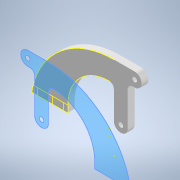
# Autodesk Inventor part: hinge
Saved by Autodesk Inventor 2020 (Build 240168000, 168)
## iProperties
Created: 2020-07-26
Part Number: hinge
Material: Generic
Document SubType Name: Modeling
Designer: Aarya
Density: 1 g/cm^3
Appearance: Default
Author: Aarya
Autodesk Inventor part; units mm, degrees
ref_plane "YZ Plane" through (0, 0, 0) normal (1, 0, 0) x (0, 1, 0)
ref_plane "XZ Plane" through (0, 0, 0) normal (0, 1, 0) x (-1, 0, 0)
ref_plane "XY Plane" through (0, 0, 0) normal (0, 0, 1) x (1, 0, 0)
sketch "Sketch1" plane through (0, 0, 0) normal (0, 0, 1) x (1, 0, 0)
  arc A0 (0, 18) -> (-18, 0.0024) centre (0, 0) ccw
  line L0 (0, 0) -> (0, -6.19)
  line L1 (0, -6.19) -> (2, -6.19)
  arc A1 (2, 30) -> (-33.6563, 0.0024) centre (2, -6.19) ccw
  line L2 (-33.6563, 0.0024) -> (-18, 0.0024)
  line L3 (3, 0) -> (3, 0)
  line L4 (6, 0) -> (32.7783, 0) construction
  line L5 (-33.6563, 0.0024) -> (-33.6563, 30.0024)
  line L6 (2, 30) -> (11, 30)
  line L7 (2, 30) -> (11, 30) construction
  line L8 (0, 0) -> (0, 3)
  line L9 (3, 3) -> (3, 3)
  line L10 (0, 3) -> (2, 3)
  line L11 (2, 6) -> (2, 16)
  line L12 (5, 3) -> (5, 3)
  line L13 (8, 6) -> (8, 22)
  arc A2 (2, 6) -> (5, 3) centre (5, 6) ccw
  arc A3 (5, 3) -> (8, 6) centre (5, 6) ccw
  arc A4 (2, 16) -> (0, 18) centre (0, 16) ccw
  arc A5 (11, 24) -> (11, 30) centre (11, 27) ccw
  line L14 (11, 24) -> (10, 24)
  arc A6 (10, 24) -> (8, 22) centre (10, 22) ccw
  circle A7 centre (5, 6) radius 1
  circle A8 centre (11, 27) radius 1
  line L15 (-33.6563, 0.0024) -> (-31.6563, 0.0024)
  line L16 (-27.1563, 0.0024) -> (-25.1563, 0.0024)
  point P0 (8, 3)
  point P1 (8, 24)
  point P2 (2, 17.8885)
  point P3 (-20.6563, 0.0024)
  dimension "d0" = 36
  dimension "d1" = 6.19
  dimension "d2" = 2
  dimension "d3" = 72.38
  dimension "d11" = 30
  dimension "d14" = 3
  dimension "d17" = 2
  dimension "d18" = 6
  dimension "d19" = 3
  dimension "d20" = 2
  dimension "d21" = 9
  dimension "d23" = 6
  dimension "d24" = 18
  dimension "d25" = 2
  dimension "d26" = 2
  dimension "d27" = 2
  dimension "d28" = 2
  dimension "d31" = 2
  constraints: 34 end point, 15 point on circle, 13 point on line, 12 tangent, 9 centre point, 7 horizontal, 4 coincident, 4 perpendicular, 3 vertical, 1 concentric
  measures "d0" diameter of A0
  measures "d1" distance of L0.start L0.end
  measures "d2" distance of L0.end L1.end
  measures "d3" diameter of A1
  measures "d11" distance of L2.start L5.end
  measures "d14" distance of L0.start L8.end
  measures "d17" distance of L8.end L10.end
  measures "d18" distance of L10.end point (8, 3)
  measures "d19" radius of A2
  measures "d20" radius of A4
  measures "d21" distance of L6.start L6.end
  measures "d23" diameter of A5
  measures "d24" distance of L13.start point (8, 24)
  measures "d25" radius of A6
  measures "d26" diameter of A7
  measures "d27" diameter of A8
  measures "d28" distance of L2.start L15.end
  measures "d31" distance of L16.start L16.end
extrude "Extrusion1" add sketch "Sketch1" against normal blind 3
sketch "Sketch2" plane through (0, 0, 0) normal (0, 0, 1) x (1, 0, 0)
  arc A0 (0.0129, 20.9952) -> (-17.9376, 1.4977) centre (-0.0001, 2.9953) ccw
  arc A1 (2, 18.9952) -> (-0.013, 20.9952) centre (-0.0001, 18.9952) ccw
  line L0 (2, 18.9952) -> (2, 16.0083)
  circle A2 centre (5, 6.9952) radius 3 projected
  circle A3 centre (5, 6.9952) radius 1 projected
  line L1 (8, 6) -> (8, 22) projected
  line L2 (-33, 2.9952) -> (-18, 2.9952) projected
  line L3 (-20, -0.0048) -> (-20, 2.9952) projected
  line L4 (-24.5, -0.0048) -> (-20, -0.0048) projected
  line L5 (-24.5, 2.9952) -> (-24.5, -0.0048) projected
  line L6 (-26.5, -0.0048) -> (-26.5, 2.9952) projected
  line L7 (-31, -0.0048) -> (-26.5, -0.0048) projected
  line L8 (-33.6563, 0.0024) -> (-18, 0.0024) projected
  arc A4 (0, 18) -> (-17.9376, 1.4977) centre (0, 0) ccw
  arc A5 (2, 16) -> (0, 18) centre (0, 16) ccw
  line L9 (2, 16) -> (2, 6) projected
  arc A6 (2, 6) -> (8, 6) centre (5, 6) ccw projected
  line L10 (8, 6) -> (8, 22) projected
  arc A7 (8, 22) -> (10, 24) centre (10, 22) ccw projected
  line L11 (10, 24) -> (11, 24) projected
  arc A8 (11, 24) -> (11, 30) centre (11, 27) ccw projected
  line L12 (11, 30) -> (2, 30) projected
  arc A9 (2, 30) -> (-33.6563, 0.0024) centre (2, -6.19) ccw projected
  circle A10 centre (11, 27) radius 1 projected
  circle A11 centre (5, 6) radius 1 projected
  line L13 (-31, 2.9952) -> (-31, -0.0048) projected
  constraints: 11 centre point, 11 point on circle, 2 end point, 1 point on line
extrude "Extrusion2" cut sketch "Sketch2" against normal blind 9.35 contours A1 L0 A5 A4 A0
sketch "Sketch4" plane through (0, 0, 0) normal (0, 0, 1) x (1, 0, 0)
  circle A0 centre (5, 6) radius 1 projected
  point P0 (0, 0)
extrude "Extrusion3" add sketch "Sketch4" against normal blind 3
sketch "Sketch5" plane through (0, 0, 0) normal (0, 0, 1) x (1, 0, 0)
  line L0 (5, 6) -> (5, 6.995) construction
  circle A0 centre (5, 6.995) radius 1
  point P0 (0, 0)
  dimension "d40" = 0.995
  dimension "d41" = 2
  constraints: 2 end point, 1 centre point, 1 coincident, 1 vertical
  measures "d40" distance of L0.start L0.end
  measures "d41" diameter of A0
extrude "Extrusion4" cut sketch "Sketch5" against normal blind 3
sketch "Sketch6" plane through (0, 0, 0) normal (0, 0, 1) x (1, 0, 0)
  arc A0 (2, 6) -> (8, 6) centre (5, 6) ccw projected
  line L0 (5, 6) -> (5, 7)
  circle A1 centre (5, 7) radius 3
  line L1 (2, 16) -> (2, 6) projected
  line L2 (8, 6) -> (8, 22) projected
  point P0 (0, 0)
  point P1 (8, 7)
  point P2 (2, 7)
  dimension "d44" = 1
  dimension "d45" = 6
  constraints: 2 end point, 1 centre point, 1 coincident, 1 vertical
  measures "d44" distance of L0.start L0.end
  measures "d45" diameter of A1
extrude "Extrusion5" cut sketch "Sketch6" against normal blind 3 contours L1 A1 L2 A0
sketch "Sketch8" plane through (0, 0, 0) normal (0, 0, 1) x (1, 0, 0)
  arc A0 (2, 30) -> (-33.6563, 0.0024) centre (2, -6.19) ccw projected
  line L0 (-33.01, 2.9759) -> (-31.01, 2.9759)
  line L1 (-31.01, 2.9759) -> (-31.01, -0.0241)
  line L2 (-31.01, -0.0241) -> (-26.5101, 0.0024)
  line L3 (-18, 0.0024) -> (-33.6563, 0.0024) projected
  line L4 (-26.5101, 0.0024) -> (-26.5278, 3.0024)
  line L5 (-26.5278, 3.0024) -> (-24.5279, 2.9759)
  line L6 (-24.5279, 2.9759) -> (-24.4163, -0.022)
  line L7 (-24.4163, -0.022) -> (-19.9163, 0.0024)
  line L8 (-19.9163, 0.0024) -> (-19.9326, 3.0024)
  line L9 (-19.9326, 3.0024) -> (-17.9328, 2.9759)
  arc A1 (2, 30) -> (-33.6563, 0.0024) centre (2, -6.19) ccw projected
  circle A2 centre (11, 27) radius 1 projected
  arc A3 (2, 7) -> (8, 7) centre (5, 7) ccw projected
  line L10 (8, 7) -> (8, 22) projected
  arc A4 (10, 24) -> (8, 22) centre (10, 22) ccw projected
  line L11 (10, 24) -> (11, 24) projected
  arc A5 (11, 24) -> (11, 30) centre (11, 27) ccw projected
  line L12 (11, 30) -> (2, 30) projected
  arc A6 (2, 30) -> (-33.6563, 0.0024) centre (2, -6.19) ccw projected
  line L13 (-33.6563, 0.0024) -> (-18, 0.0024) projected
  arc A7 (-17.9376, 1.4977) -> (-18, 0.0024) centre (0, 0) ccw projected
  arc A8 (0.0129, 20.9952) -> (-17.9376, 1.4977) centre (-0.0001, 2.9953) ccw projected
  arc A9 (2, 18.9952) -> (0.0129, 20.9952) centre (-0.0001, 18.9952) ccw projected
  line L14 (2, 18.9952) -> (2, 16.0083) projected
  arc A10 (2, 16) -> (2, 16.0083) centre (0, 16) ccw projected
  line L15 (2, 16) -> (2, 7) projected
  circle A11 centre (5, 6.995) radius 1 projected
  point P0 (-18, 2.9768)
  point P1 (-31.01, 0.0024)
  point P2 (-24.4172, 0.0024)
  dimension "d48" = 2
  dimension "d49" = 3
  dimension "d50" = 4.5
  dimension "d51" = 3
  dimension "d52" = 2
  dimension "d53" = 3
  dimension "d54" = 4.5
  dimension "d55" = 3
  dimension "d56" = 2
  constraints: 18 end point, 4 point on line, 3 perpendicular, 1 horizontal, 1 point on circle
  measures "d48" distance of L0.start L0.end
  measures "d49" distance of L0.end L1.end
  measures "d50" distance of L1.end L2.end
  measures "d51" distance of L2.end L4.end
  measures "d52" distance of L4.end L5.end
  measures "d53" distance of L5.end L6.end
  measures "d54" distance of L6.end L7.end
  measures "d55" distance of L7.end L8.end
  measures "d56" distance of L8.end L9.end
extrude "Extrusion6" cut sketch "Sketch8" against normal blind 3 contours L0 L1 L3 A0 | L4 L5 L6 L3 | L8 L9 A8 A7 L3
body "Solid1"
